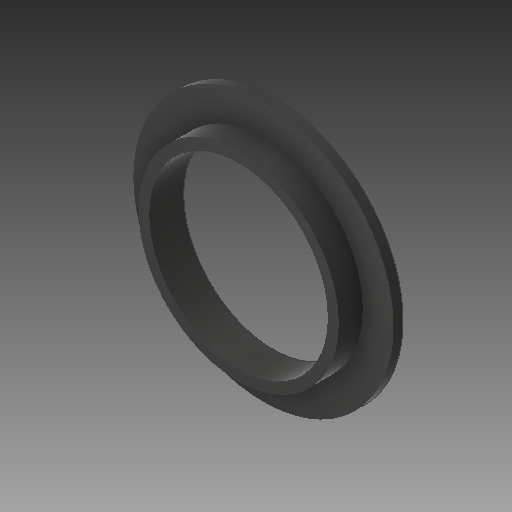
# Autodesk Inventor part: オイレスフランジ付き18202.5
Saved by Autodesk Inventor 2020 (Build 240168000, 168)
## iProperties
Created: 2018-11-18
Part Number: オイレスフランジ付き18202.5
Material: アセタール樹脂、黒
Document SubType Name: Modeling
Designer: 雪村
Density: 1.425 g/cm^3
Appearance: 滑らか - 黒
Mass: 0.606602 g
Surface Area: 9.89602 cm^2
Volume: 0.425686 cm^3
Author: 雪村
Autodesk Inventor part; units mm, degrees
ref_plane "YZ Plane" through (0, 0, 0) normal (1, 0, 0) x (0, 1, 0)
ref_plane "XZ Plane" through (0, 0, 0) normal (0, 1, 0) x (-1, 0, 0)
ref_plane "XY Plane" through (0, 0, 0) normal (0, 0, 1) x (1, 0, 0)
sketch "スケッチ1" plane through (0, 0, 0) normal (0, 0, 1) x (1, 0, 0)
  circle A0 centre (0, 0) radius 9
  circle A1 centre (0, 0) radius 10
  dimension "d0" = 18
  dimension "d1" = 20
  constraints: 2 centre point, 2 coincident
  measures "d0" diameter of A0
  measures "d1" diameter of A1
extrude "押し出し1" add sketch "スケッチ1" along normal blind 2.5
sketch "スケッチ2" plane through (0, 0, 0) normal (0, 0, -1) x (-1, 0, 0)
  circle A0 centre (0, 0) radius 9 projected
  circle A1 centre (0, 0) radius 10 projected
  circle A2 centre (0, 0) radius 13
  dimension "d4" = 26
  constraints: 1 centre point, 1 coincident
  measures "d4" diameter of A2
extrude "押し出し2" add sketch "スケッチ2" along normal blind 1 contours A1 | A2
